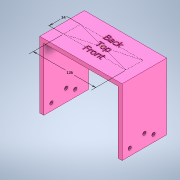
# Autodesk Inventor part: squareBracketForLowerGarage
Saved by Autodesk Inventor 2022.1 (Build 261234020, 234B)
## iProperties
Created: 2021-10-20
Part Number: squareBracketForLowerGarage
Material: PC/ABS Plastic
Document SubType Name: Modeling
Designer: robst
Density: 0.357273 g/cm^3
Appearance: Pink
Author: robst
Autodesk Inventor part; units mm, degrees
ref_plane "YZ Plane" through (0, 0, 0) normal (1, 0, 0) x (0, 1, 0)
ref_plane "XZ Plane" through (0, 0, 0) normal (0, 1, 0) x (-1, 0, 0)
ref_plane "XY Plane" through (0, 0, 0) normal (0, 0, 1) x (1, 0, 0)
sketch "Sketch47" plane through (0, 0, 0) normal (0, 1, 0) x (-1, 0, 0)
  line L0 (83, 45) -> (-83, 45)
  line L1 (-83, 45) -> (-83, -45)
  line L2 (-83, -45) -> (83, -45)
  line L3 (83, -45) -> (83, 45)
  line L4 (83, 45) -> (-83, -45) construction
  line L5 (-83, 45) -> (83, -45) construction
  point P0 (0, 0)
  dimension "d218" = 90
  dimension "d219" = 166
  constraints: 12 end point, 2 midpoint, 2 parallel, 1 horizontal, 1 perpendicular
  measures "d218" distance of L2.end L0.start
  measures "d219" distance of L1.end L2.end
extrude "Extrusion22" add sketch "Sketch47" along normal blind 8
sketch "Sketch48" plane through (0, 0, 0) normal (0, -1, 0) x (1, 0, 0)
  line L0 (-83, -45) -> (-83, 45) projected
  line L1 (83, -45) -> (-83, -45) projected
  line L2 (-83, 45) -> (-75, 45)
  line L3 (-75, 45) -> (-75, -45)
  line L4 (-75, -45) -> (-83, -45)
  line L5 (-83, -45) -> (-83, 45)
  line L6 (83, 45) -> (83, -45) projected
  line L7 (83, 45) -> (75, 45)
  line L8 (75, 45) -> (75, -45)
  line L9 (75, -45) -> (83, -45)
  line L10 (83, -45) -> (83, 45)
  point P0 (0, 0)
  point P1 (75, -45)
  dimension "d222" = 8
  dimension "d223" = 8
  constraints: 16 end point, 4 parallel, 2 horizontal, 2 perpendicular, 2 point on line
  measures "d222" distance between parallel lines of L3 L0
  measures "d223" distance between parallel lines of L8 L6
extrude "Extrusion23" add sketch "Sketch48" along normal blind 126
sketch "Sketch49" plane through (0, 8, 0) normal (0, 1, 0) x (1, 0, 0)
  line L0 (-83, 45) -> (-83, -45) construction
  line L1 (-83, 0) -> (83, 0) construction
  line L2 (83, -45) -> (83, 45) construction
  spline S0 degree 2 poles (-7.7553, 18.6856) (-7.7553, 17.7909) (-8.436, 16.4198) (-9, 15.9724) knots 0 0 0 1 2 2 2
  spline S1 degree 2 poles (-9, 15.9724) (-9.6807, 15.4473) (-11.2269, 15) (-12.4522, 15) knots 0 0 0 1 2 2 2
  line L3 (-12.4522, 15) -> (-15.8947, 15)
  line L4 (-15.8947, 15) -> (-15.8947, 27)
  line L5 (-15.8947, 27) -> (-12.7147, 27)
  spline S2 degree 2 poles (-12.7147, 27) (-11.4311, 27) (-10.1475, 26.8347) (-9.564, 26.5138) knots 0 0 0 1 2 2 2
  spline S3 degree 2 poles (-9.564, 26.5138) (-8.9125, 26.1734) (-8.3193, 25.0551) (-8.3193, 24.2966) knots 0 0 0 1 2 2 2
  spline S4 degree 2 poles (-8.3193, 24.2966) (-8.3193, 23.4506) (-9.2139, 22.1086) (-10.0016, 21.7293) knots 0 0 0 1 2 2 2
  line L6 (-10.0016, 21.7293) -> (-10.0016, 21.671)
  spline S5 degree 2 poles (-10.0016, 21.671) (-8.9319, 21.3793) (-7.7553, 19.8331) (-7.7553, 18.6856) knots 0 0 0 1 2 2 2
  spline S6 degree 2 poles (-9.4182, 18.6175) (-9.4182, 19.2982) (-9.8071, 20.1734) (-10.3906, 20.4846) knots 0 0 0 1 2 2 2
  spline S7 degree 2 poles (-10.3906, 20.4846) (-10.7699, 20.6791) (-11.6645, 20.7958) (-12.4911, 20.7958) knots 0 0 0 1 2 2 2
  line L7 (-12.4911, 20.7958) -> (-14.2998, 20.7958)
  line L8 (-14.2998, 20.7958) -> (-14.2998, 16.3614)
  line L9 (-14.2998, 16.3614) -> (-13.0065, 16.3614)
  spline S8 degree 2 poles (-13.0065, 16.3614) (-11.9562, 16.3614) (-10.7504, 16.5559) (-10.2836, 16.8671) knots 0 0 0 1 2 2 2
  spline S9 degree 2 poles (-10.2836, 16.8671) (-9.8363, 17.188) (-9.4182, 17.9854) (-9.4182, 18.6175) knots 0 0 0 1 2 2 2
  spline S10 degree 2 poles (-9.9822, 24.0729) (-9.9822, 24.5008) (-10.2739, 25.1426) (-10.5948, 25.3274) knots 0 0 0 1 2 2 2
  spline S11 degree 2 poles (-10.5948, 25.3274) (-10.9838, 25.5413) (-11.9271, 25.6386) (-12.7731, 25.6386) knots 0 0 0 1 2 2 2
  line L10 (-12.7731, 25.6386) -> (-14.2998, 25.6386)
  line L11 (-14.2998, 25.6386) -> (-14.2998, 22.128)
  line L12 (-14.2998, 22.128) -> (-12.4911, 22.128)
  spline S12 degree 2 poles (-12.4911, 22.128) (-11.7423, 22.128) (-11.0324, 22.2836) (-10.6532, 22.5267) knots 0 0 0 1 2 2 2
  spline S13 degree 2 poles (-10.6532, 22.5267) (-10.2836, 22.7601) (-9.9822, 23.5089) (-9.9822, 24.0729) knots 0 0 0 1 2 2 2
  spline S14 degree 2 poles (-1.269, 15.953) (-1.4538, 15.8169) (-2.0762, 15.3306) (-2.3679, 15.1848) knots 0 0 0 1 2 2 2
  spline S15 degree 2 poles (-2.3679, 15.1848) (-2.7666, 14.9708) (-3.5154, 14.7472) (-4.1961, 14.7472) knots 0 0 0 1 2 2 2
  spline S16 degree 2 poles (-4.1961, 14.7472) (-4.7504, 14.7472) (-5.752, 15.1653) (-6.1313, 15.5446) knots 0 0 0 1 2 2 2
  spline S17 degree 2 poles (-6.1313, 15.5446) (-6.4911, 15.9141) (-6.9287, 17.0032) (-6.9287, 17.6062) knots 0 0 0 1 2 2 2
  spline S18 degree 2 poles (-6.9287, 17.6062) (-6.9287, 18.5397) (-6.141, 19.8622) (-5.2853, 20.2415) knots 0 0 0 1 2 2 2
  spline S19 degree 2 poles (-5.2853, 20.2415) (-4.5267, 20.5916) (-2.4652, 20.8541) (-1.269, 20.9222) knots 0 0 0 1 2 2 2
  line L13 (-1.269, 20.9222) -> (-1.269, 21.2139)
  spline S20 degree 2 poles (-1.269, 21.2139) (-1.269, 21.7391) (-1.59, 22.3906) (-1.8817, 22.5754) knots 0 0 0 1 2 2 2
  spline S21 degree 2 poles (-1.8817, 22.5754) (-2.1734, 22.7601) (-3.0097, 22.8768) (-3.4571, 22.8768) knots 0 0 0 1 2 2 2
  spline S22 degree 2 poles (-3.4571, 22.8768) (-3.9822, 22.8768) (-5.4019, 22.5656) (-6.1118, 22.2642) knots 0 0 0 1 2 2 2
  line L14 (-6.1118, 22.2642) -> (-6.1994, 22.2642)
  line L15 (-6.1994, 22.2642) -> (-6.1994, 23.8104)
  spline S23 degree 2 poles (-6.1994, 23.8104) (-5.7812, 23.9271) (-4.2156, 24.2188) (-3.4473, 24.2188) knots 0 0 0 1 2 2 2
  spline S24 degree 2 poles (-3.4473, 24.2188) (-2.5138, 24.2188) (-1.2399, 23.9271) (-0.7342, 23.5478) knots 0 0 0 1 2 2 2
  spline S25 degree 2 poles (-0.7342, 23.5478) (-0.2382, 23.1783) (0.248, 22.0016) (0.248, 21.1556) knots 0 0 0 1 2 2 2
  line L16 (0.248, 21.1556) -> (0.248, 15)
  line L17 (0.248, 15) -> (-1.269, 15)
  line L18 (-1.269, 15) -> (-1.269, 15.953)
  line L19 (-1.269, 17.2172) -> (-1.269, 19.7164)
  spline S26 degree 2 poles (-1.269, 19.7164) (-1.8136, 19.6677) (-3.4571, 19.5024) (-3.9724, 19.3468) knots 0 0 0 1 2 2 2
  spline S27 degree 2 poles (-3.9724, 19.3468) (-4.5754, 19.1621) (-5.363, 18.3938) (-5.363, 17.7131) knots 0 0 0 1 2 2 2
  spline S28 degree 2 poles (-5.363, 17.7131) (-5.363, 16.9352) (-4.4878, 16.1475) (-3.6515, 16.1475) knots 0 0 0 1 2 2 2
  spline S29 degree 2 poles (-3.6515, 16.1475) (-2.9417, 16.1475) (-1.7747, 16.7601) (-1.269, 17.2172) knots 0 0 0 1 2 2 2
  spline S30 degree 2 poles (5.9562, 14.7958) (5.0227, 14.7958) (3.4765, 15.3695) (2.9222, 15.953) knots 0 0 0 1 2 2 2
  spline S31 degree 2 poles (2.9222, 15.953) (2.3679, 16.5267) (1.7553, 18.2966) (1.7553, 19.483) knots 0 0 0 1 2 2 2
  spline S32 degree 2 poles (1.7553, 19.483) (1.7553, 20.6694) (2.3874, 22.4003) (2.9222, 22.9838) knots 0 0 0 1 2 2 2
  spline S33 degree 2 poles (2.9222, 22.9838) (3.4571, 23.577) (5.0421, 24.2091) (5.9562, 24.2091) knots 0 0 0 1 2 2 2
  spline S34 degree 2 poles (5.9562, 24.2091) (6.6953, 24.2091) (8.0762, 23.7909) (8.611, 23.5186) knots 0 0 0 1 2 2 2
  line L20 (8.611, 23.5186) -> (8.611, 21.8169)
  line L21 (8.611, 21.8169) -> (8.5235, 21.8169)
  spline S35 degree 2 poles (8.5235, 21.8169) (8.3582, 21.953) (7.8525, 22.3031) (7.4927, 22.4878) knots 0 0 0 1 2 2 2
  spline S36 degree 2 poles (7.4927, 22.4878) (7.1718, 22.6434) (6.316, 22.8865) (5.9271, 22.8865) knots 0 0 0 1 2 2 2
  spline S37 degree 2 poles (5.9271, 22.8865) (4.7504, 22.8865) (3.3209, 21.107) (3.3209, 19.483) knots 0 0 0 1 2 2 2
  spline S38 degree 2 poles (3.3209, 19.483) (3.3209, 17.8979) (4.7018, 16.1183) (5.9271, 16.1183) knots 0 0 0 1 2 2 2
  spline S39 degree 2 poles (5.9271, 16.1183) (6.6661, 16.1183) (8.0081, 16.731) (8.5235, 17.2075) knots 0 0 0 1 2 2 2
  line L22 (8.5235, 17.2075) -> (8.611, 17.2075)
  line L23 (8.611, 17.2075) -> (8.611, 15.5057)
  spline S40 degree 2 poles (8.611, 15.5057) (8.3874, 15.3987) (7.7066, 15.0972) (7.4344, 15.0292) knots 0 0 0 1 2 2 2
  spline S41 degree 2 poles (7.4344, 15.0292) (7.0454, 14.9125) (6.4327, 14.7958) (5.9562, 14.7958) knots 0 0 0 1 2 2 2
  line L24 (17.4506, 15) -> (15.4571, 15)
  line L25 (15.4571, 15) -> (12.1118, 19.3468)
  line L26 (12.1118, 19.3468) -> (11.5089, 18.7634)
  line L27 (11.5089, 18.7634) -> (11.5089, 15)
  line L28 (11.5089, 15) -> (9.9919, 15)
  line L29 (9.9919, 15) -> (9.9919, 27.5348)
  line L30 (9.9919, 27.5348) -> (11.5089, 27.5348)
  line L31 (11.5089, 27.5348) -> (11.5089, 20.2026)
  line L32 (11.5089, 20.2026) -> (15.0681, 24.0049)
  line L33 (15.0681, 24.0049) -> (16.9546, 24.0049)
  line L34 (16.9546, 24.0049) -> (13.2593, 20.2415)
  line L35 (13.2593, 20.2415) -> (17.4506, 15)
  line L36 (-9.8412, -4.5635) -> (-9.8412, 6.0168)
  line L37 (-9.8412, 6.0168) -> (-13.8671, 6.0168)
  line L38 (-13.8671, 6.0168) -> (-13.8671, 7.4365)
  line L39 (-13.8671, 7.4365) -> (-4.2204, 7.4365)
  line L40 (-4.2204, 7.4365) -> (-4.2204, 6.0168)
  line L41 (-4.2204, 6.0168) -> (-8.2464, 6.0168)
  line L42 (-8.2464, 6.0168) -> (-8.2464, -4.5635)
  line L43 (-8.2464, -4.5635) -> (-9.8412, -4.5635)
  spline S42 degree 2 poles (4.2885, -0.061) (4.2885, -2.3366) (2.1005, -4.8163) (0.2723, -4.8163) knots 0 0 0 1 2 2 2
  spline S43 degree 2 poles (0.2723, -4.8163) (-1.6045, -4.8163) (-3.7536, -2.2588) (-3.7536, -0.061) knots 0 0 0 1 2 2 2
  spline S44 degree 2 poles (-3.7536, -0.061) (-3.7536, 2.195) (-1.5365, 4.6942) (0.2723, 4.6942) knots 0 0 0 1 2 2 2
  spline S45 degree 2 poles (0.2723, 4.6942) (2.1005, 4.6942) (4.2885, 2.2048) (4.2885, -0.061) knots 0 0 0 1 2 2 2
  spline S46 degree 2 poles (2.7229, -0.061) (2.7229, 1.6894) (1.4489, 3.3911) (0.2723, 3.3911) knots 0 0 0 1 2 2 2
  spline S47 degree 2 poles (0.2723, 3.3911) (-0.9044, 3.3911) (-2.188, 1.6894) (-2.188, -0.061) knots 0 0 0 1 2 2 2
  spline S48 degree 2 poles (-2.188, -0.061) (-2.188, -1.7628) (-0.9044, -3.5132) (0.2723, -3.5132) knots 0 0 0 1 2 2 2
  spline S49 degree 2 poles (0.2723, -3.5132) (1.4392, -3.5132) (2.7229, -1.792) (2.7229, -0.061) knots 0 0 0 1 2 2 2
  spline S50 degree 2 poles (13.3906, 0.1821) (13.3906, -2.074) (11.2415, -4.7385) (9.5981, -4.7385) knots 0 0 0 1 2 2 2
  spline S51 degree 2 poles (9.5981, -4.7385) (8.9271, -4.7385) (7.8963, -4.4273) (7.3614, -4.1064) knots 0 0 0 1 2 2 2
  line L44 (7.3614, -4.1064) -> (7.3614, -7.8795)
  line L45 (7.3614, -7.8795) -> (5.8444, -7.8795)
  line L46 (5.8444, -7.8795) -> (5.8444, 4.4414)
  line L47 (5.8444, 4.4414) -> (7.3614, 4.4414)
  line L48 (7.3614, 4.4414) -> (7.3614, 3.4981)
  spline S52 degree 2 poles (7.3614, 3.4981) (7.9254, 4.0135) (9.3063, 4.6942) (10.1135, 4.6942) knots 0 0 0 1 2 2 2
  spline S53 degree 2 poles (10.1135, 4.6942) (11.6596, 4.6942) (13.3906, 2.2437) (13.3906, 0.1821) knots 0 0 0 1 2 2 2
  spline S54 degree 2 poles (11.825, 0.007) (11.825, 1.5532) (10.8428, 3.255) (9.7439, 3.255) knots 0 0 0 1 2 2 2
  spline S55 degree 2 poles (9.7439, 3.255) (9.1021, 3.255) (7.8963, 2.6813) (7.3614, 2.2339) knots 0 0 0 1 2 2 2
  line L49 (7.3614, 2.2339) -> (7.3614, -2.8811)
  spline S56 degree 2 poles (7.3614, -2.8811) (7.9546, -3.1632) (8.8006, -3.3771) (9.3452, -3.3771) knots 0 0 0 1 2 2 2
  spline S57 degree 2 poles (9.3452, -3.3771) (10.5219, -3.3771) (11.825, -1.6461) (11.825, 0.007) knots 0 0 0 1 2 2 2
  line L50 (-10.7261, -13.5467) -> (-16.3079, -13.5467)
  line L51 (-16.3079, -13.5467) -> (-16.3079, -16.9308)
  line L52 (-16.3079, -16.9308) -> (-10.9595, -16.9308)
  line L53 (-10.9595, -16.9308) -> (-10.9595, -18.3506)
  line L54 (-10.9595, -18.3506) -> (-16.3079, -18.3506)
  line L55 (-16.3079, -18.3506) -> (-16.3079, -24.127)
  line L56 (-16.3079, -24.127) -> (-17.9028, -24.127)
  line L57 (-17.9028, -24.127) -> (-17.9028, -12.127)
  line L58 (-17.9028, -12.127) -> (-10.7261, -12.127)
  line L59 (-10.7261, -12.127) -> (-10.7261, -13.5467)
  line L60 (-4.6386, -16.7461) -> (-4.7164, -16.7461)
  spline S58 degree 2 poles (-4.7164, -16.7461) (-4.8914, -16.6975) (-5.2707, -16.678) (-5.5332, -16.678) knots 0 0 0 1 2 2 2
  spline S59 degree 2 poles (-5.5332, -16.678) (-6.1459, -16.678) (-7.3517, -17.2128) (-7.8963, -17.738) knots 0 0 0 1 2 2 2
  line L61 (-7.8963, -17.738) -> (-7.8963, -24.127)
  line L62 (-7.8963, -24.127) -> (-9.4133, -24.127)
  line L63 (-9.4133, -24.127) -> (-9.4133, -15.1221)
  line L64 (-9.4133, -15.1221) -> (-7.8963, -15.1221)
  line L65 (-7.8963, -15.1221) -> (-7.8963, -16.4641)
  spline S60 degree 2 poles (-7.8963, -16.4641) (-7.0697, -15.725) (-5.8347, -15.1221) (-5.2512, -15.1221) knots 0 0 0 1 2 2 2
  spline S61 degree 2 poles (-5.2512, -15.1221) (-5.0178, -15.1221) (-4.7844, -15.1415) (-4.6386, -15.1707) knots 0 0 0 1 2 2 2
  line L66 (-4.6386, -15.1707) -> (-4.6386, -16.7461)
  spline S62 degree 2 poles (3.9384, -19.6245) (3.9384, -21.9) (1.7504, -24.3798) (-0.0778, -24.3798) knots 0 0 0 1 2 2 2
  spline S63 degree 2 poles (-0.0778, -24.3798) (-1.9546, -24.3798) (-4.1037, -21.8223) (-4.1037, -19.6245) knots 0 0 0 1 2 2 2
  spline S64 degree 2 poles (-4.1037, -19.6245) (-4.1037, -17.3684) (-1.8865, -14.8693) (-0.0778, -14.8693) knots 0 0 0 1 2 2 2
  spline S65 degree 2 poles (-0.0778, -14.8693) (1.7504, -14.8693) (3.9384, -17.3587) (3.9384, -19.6245) knots 0 0 0 1 2 2 2
  spline S66 degree 2 poles (2.3728, -19.6245) (2.3728, -17.8741) (1.0989, -16.1723) (-0.0778, -16.1723) knots 0 0 0 1 2 2 2
  spline S67 degree 2 poles (-0.0778, -16.1723) (-1.2545, -16.1723) (-2.5381, -17.8741) (-2.5381, -19.6245) knots 0 0 0 1 2 2 2
  spline S68 degree 2 poles (-2.5381, -19.6245) (-2.5381, -21.3263) (-1.2545, -23.0767) (-0.0778, -23.0767) knots 0 0 0 1 2 2 2
  spline S69 degree 2 poles (-0.0778, -23.0767) (1.0891, -23.0767) (2.3728, -21.3555) (2.3728, -19.6245) knots 0 0 0 1 2 2 2
  line L67 (12.564, -24.127) -> (11.047, -24.127)
  line L68 (11.047, -24.127) -> (11.047, -18.9924)
  spline S70 degree 2 poles (11.047, -18.9924) (11.047, -18.3701) (10.9303, -17.3004) (10.7553, -16.9795) knots 0 0 0 1 2 2 2
  spline S71 degree 2 poles (10.7553, -16.9795) (10.5705, -16.6391) (9.9092, -16.3085) (9.3452, -16.3085) knots 0 0 0 1 2 2 2
  spline S72 degree 2 poles (9.3452, -16.3085) (8.7812, -16.3085) (7.5851, -16.9114) (7.0113, -17.3976) knots 0 0 0 1 2 2 2
  line L69 (7.0113, -17.3976) -> (7.0113, -24.127)
  line L70 (7.0113, -24.127) -> (5.4943, -24.127)
  line L71 (5.4943, -24.127) -> (5.4943, -15.1221)
  line L72 (5.4943, -15.1221) -> (7.0113, -15.1221)
  line L73 (7.0113, -15.1221) -> (7.0113, -16.1237)
  spline S73 degree 2 poles (7.0113, -16.1237) (7.6921, -15.5111) (9.0049, -14.8693) (9.7439, -14.8693) knots 0 0 0 1 2 2 2
  spline S74 degree 2 poles (9.7439, -14.8693) (11.0665, -14.8693) (12.564, -16.6197) (12.564, -18.2825) knots 0 0 0 1 2 2 2
  line L74 (12.564, -18.2825) -> (12.564, -24.127)
  spline S75 degree 2 poles (17.4165, -24.302) (16.1815, -24.302) (14.7909, -22.8919) (14.7909, -21.3652) knots 0 0 0 1 2 2 2
  line L75 (14.7909, -21.3652) -> (14.7909, -16.3765)
  line L76 (14.7909, -16.3765) -> (13.7699, -16.3765)
  line L77 (13.7699, -16.3765) -> (13.7699, -15.1221)
  line L78 (13.7699, -15.1221) -> (14.7909, -15.1221)
  line L79 (14.7909, -15.1221) -> (14.7909, -12.5354)
  line L80 (14.7909, -12.5354) -> (16.3079, -12.5354)
  line L81 (16.3079, -12.5354) -> (16.3079, -15.1221)
  line L82 (16.3079, -15.1221) -> (19.0989, -15.1221)
  line L83 (19.0989, -15.1221) -> (19.0989, -16.3765)
  line L84 (19.0989, -16.3765) -> (16.3079, -16.3765)
  line L85 (16.3079, -16.3765) -> (16.3079, -20.665)
  spline S76 degree 2 poles (16.3079, -20.665) (16.3079, -21.3458) (16.3566, -22.0945) (16.5219, -22.4154) knots 0 0 0 1 2 2 2
  spline S77 degree 2 poles (16.5219, -22.4154) (16.658, -22.6975) (17.2707, -22.9795) (17.7958, -22.9795) knots 0 0 0 1 2 2 2
  spline S78 degree 2 poles (17.7958, -22.9795) (18.1653, -22.9795) (18.8558, -22.7558) (19.0113, -22.6877) knots 0 0 0 1 2 2 2
  line L86 (19.0113, -22.6877) -> (19.0989, -22.6877)
  line L87 (19.0989, -22.6877) -> (19.0989, -24.0492)
  spline S79 degree 2 poles (19.0989, -24.0492) (18.671, -24.1658) (17.7958, -24.302) (17.4165, -24.302) knots 0 0 0 1 2 2 2
  point P0 (0, 0)
  constraints: 2 end point, 2 midpoint, 1 horizontal
emboss "Emboss1" sketch "Sketch49" operation cut depth 1 direction (0, -1, 0)
sketch "Sketch51" plane through (-83, 8, -45) normal (-1, 0, 0) x (0, 0, 1)
  line L0 (0, -134) -> (0, 0) construction
  line L1 (0, -109) -> (90, -109) construction
  line L2 (90, 0) -> (90, -134) construction
  line L3 (0, -134) -> (90, -134) projected
  point P0 (45, -8)
  point P1 (0, -142)
  point P2 (90, -142)
  point P3 (45, -109)
  dimension "d230" = 25
  constraints: 2 end point, 2 point on line, 1 horizontal, 1 midpoint
  measures "d230" distance between parallel lines of L1 L3
hole "Hole6" at (-83, -101, 0) direction (1, 0, 0) diameter 6.756 end through all clearance for "Flat Head Machine Screw (82)" size "1/4" standard "Ansi Unified Screw Threads"
sketch "Sketch52" plane through (-83, 8, -45) normal (-1, 0, 0) x (0, 0, 1)
  line L0 (0, -134) -> (90, -134) projected
  line L1 (0, -134) -> (0, 0) projected
  line L2 (90, -134) -> (90, 0) projected
  line L3 (0, -8) -> (0, -134) construction
  line L4 (0, -120) -> (90, -120) construction
  line L5 (90, -8) -> (90, -134) construction
  circle A0 centre (45, -109) radius 3.378 construction
  line L6 (45, -142) -> (45, -109) construction
  point P0 (45, -8)
  point P1 (26.65, -120)
  point P2 (74.65, -120)
  dimension "d238" = 14
  dimension "d239" = 18.35
  dimension "d240" = 29.65
  constraints: 4 end point, 4 point on line, 1 perpendicular, 1 vertical
  measures "d238" distance between parallel lines of L4 L0
  measures "d239" distance from line of point (26.65, -120) L6
  measures "d240" distance from line of point (74.65, -120) L6
hole "Hole7" at (-83, -112, -18.35) at (-83, -112, 29.65) direction (1, 0, 0) diameter 6.756 end through all clearance for "Hex Machine Screw" size "1/4" standard "Ansi Unified Screw Threads"
sketch "Sketch53" plane through (0, 8, 0) normal (0, 1, 0) x (1, 0, 0)
  line L0 (-63, -17) -> (63, -17) construction
  line L1 (63, -17) -> (63, 17) construction
  line L2 (63, 17) -> (-63, 17) construction
  line L3 (-63, 17) -> (-63, -17) construction
  line L4 (-63, -17) -> (63, 17) construction
  line L5 (63, -17) -> (-63, 17) construction
  point P0 (0, 0)
  dimension "d248" = 34
  dimension "d249" = 126
  constraints: 12 end point, 2 midpoint, 2 parallel, 1 horizontal, 1 perpendicular
  measures "d248" distance of L2.end L0.start
  measures "d249" distance of L0.start L0.end
equation "\"d218\" = widthOfBracket"
equation "\"d219\" = widthOfUBolt + 2 * sideWallThickness"
equation "\"d220\" = topWallThickness"
equation "\"d222\" = sideWallThickness"
equation "\"d223\" = sideWallThickness"
equation "\"d224\" = sideHeightFromBottom"
equation "\"wallThickness\" = 8"
equation "\"widthOfBracket\" = 90"
equation "\"twoByFourWidth\" = 40.64"
equation "\"twoByFourDepth\" = 84.1375"
equation "\"azimuth\" = -15deg"
equation "\"elevation\" = 20deg"
equation "\"depthOfExtrusionForMatingToLowerHalf\" = 12.5"
equation "\"depthForWasherForMatingToCase\" = 14"
equation "\"topWallThickness\" = 8"
equation "\"widthOfCase\" = 149"
equation "\"sideWallThickness\" = 8"
equation "\"caseHeight\" = 125"
equation "\"bottomWallThickness\" = 8"
equation "\"widthOfUBolt\" = 150"
equation "\"sideHeightFromBottom\" = 126"
body "Solid3"
